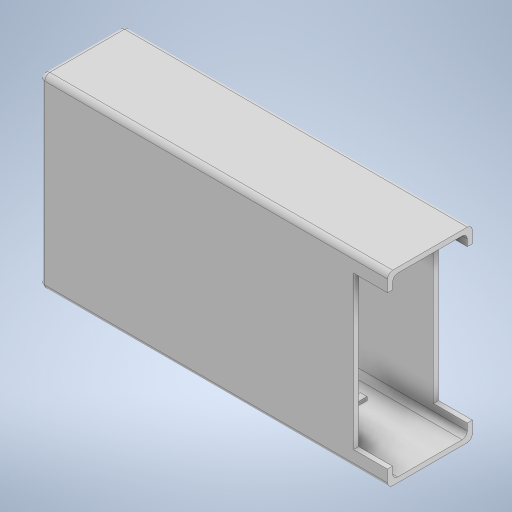
# Autodesk Inventor part: np2_headstage_box_v2
Saved by Autodesk Inventor 2023.3 (Build 273359000, 359)
## iProperties
Created: 2023-11-29
Part Number: np2_headstage_box_v2
Material: Generic
Document SubType Name: Modeling
Designer: mmelin
Density: 1 g/cm^3
Appearance: Default
Author: mmelin
Autodesk Inventor part; units mm, degrees
ref_plane "YZ Plane" through (0, 0, 0) normal (1, 0, 0) x (0, 1, 0)
ref_plane "XZ Plane" through (0, 0, 0) normal (0, 1, 0) x (-1, 0, 0)
ref_plane "XY Plane" through (0, 0, 0) normal (0, 0, 1) x (1, 0, 0)
sketch "Sketch1" plane through (0, 0, 0) normal (0, 0, 1) x (1, 0, 0)
  line L0 (0, 0) -> (18.5, 0)
  line L1 (18.5, 0) -> (18.5, -0.3)
  line L2 (18.5, -0.3) -> (0, -0.3)
  line L3 (0, -0.3) -> (0, 0)
  line L4 (18.5, 10.7) -> (0, 10.7)
  line L5 (0, 10.7) -> (0, 10.4)
  line L6 (0, 10.4) -> (18.5, 10.4)
  line L7 (18.5, 10.4) -> (18.5, 10.7)
  line L8 (0, 10.7) -> (0.3, 10.7)
  line L9 (0.3, 10.7) -> (0.3, -0.3)
  line L10 (0.3, -0.3) -> (0, -0.3)
  line L11 (0, -0.3) -> (0, 10.7)
  point P0 (0.3, 0)
  point P1 (0.3, 10.4)
  dimension "d0" = 0.3
  dimension "d1" = 18.5
  dimension "d2" = 10.4
  dimension "d3" = 0.3
  constraints: 24 end point, 8 parallel, 3 horizontal, 3 perpendicular, 1 collinear, 1 point on line
  measures "d0" distance of L0.end L1.end
  measures "d1" distance of L1.end L2.end
  measures "d2" distance between parallel lines of L0 L6
  measures "d3" distance between parallel lines of L11 L9
extrude "Extrusion1" add sketch "Sketch1" along normal blind 5
sketch "Sketch2" plane through (0.3, 0, 0) normal (1, 0, 0) x (0, 0, -1)
  line L0 (-5, 0) -> (-5, 10.4) projected
  line L1 (0, 0) -> (-5, 0) projected
  line L2 (-5, 10.4) -> (-4.7, 10.4)
  line L3 (-4.7, 10.4) -> (-4.7, 0)
  line L4 (-4.7, 0) -> (-5, 0)
  line L5 (-5, 0) -> (-5, 10.4)
  line L6 (0, 10.4) -> (-5, 10.4) projected
  line L7 (0, 0) -> (-0.3, 0)
  line L8 (-0.3, 0) -> (-0.3, 10.4)
  line L9 (-0.3, 10.4) -> (0, 10.4)
  line L10 (0, 10.4) -> (0, 0)
  point P0 (-0.3, 0)
  dimension "d6" = 0.3
  dimension "d7" = 0.3
  constraints: 16 end point, 4 parallel, 2 horizontal, 2 perpendicular, 2 point on line
  measures "d6" distance between parallel lines of L10 L8
  measures "d7" distance between parallel lines of L0 L3
extrude "Extrusion2" add sketch "Sketch2" along normal up to surface (18.2 mm away) contours L0 L2 L3 L1 | L8 L6 L10 L1
sketch "Sketch3" plane through (0, -0.3, 0) normal (-1, 0, 0) x (0, 0, 1)
  line L0 (0.9, 5.2) -> (3.2, 5.2)
  line L1 (3.2, 5.2) -> (3.2, 7.5)
  line L2 (3.2, 7.5) -> (0.9, 7.5)
  line L3 (0.9, 7.5) -> (0.9, 5.2)
  line L4 (5, 11) -> (5, 0) projected
  line L5 (0, 11) -> (5, 11) projected
  point P0 (0, 0.3)
  dimension "d10" = 2.3
  dimension "d11" = 2.3
  dimension "d12" = 1.8
  dimension "d13" = 3.5
  constraints: 8 end point, 2 parallel, 1 horizontal, 1 perpendicular
  measures "d10" distance of L2.end L0.start
  measures "d11" distance of L1.end L2.end
  measures "d12" distance between parallel lines of L4 L1
  measures "d13" distance between parallel lines of L5 L2
extrude "Extrusion3" cut sketch "Sketch3" against normal up to surface (0.3 mm away)
sketch "Sketch4" plane through (0.3, 0, 0.3) normal (0, 1, 0) x (1, 0, 0)
  line L0 (15, -3.3) -> (15.4, -3.3)
  line L1 (15.4, -3.3) -> (15.4, -1.1)
  line L2 (15.4, -1.1) -> (15, -1.1)
  line L3 (15, -1.1) -> (15, -3.3)
  line L4 (0, 0) -> (0, -4.4) projected
  line L5 (15.4, -3.3) -> (15.4, -4.4) construction
  line L6 (0, -4.4) -> (18.2, -4.4) construction
  line L7 (15.4, -1.1) -> (15.4, 0) construction
  line L8 (18.2, 0) -> (0, 0) construction
  point P0 (-0.3, 0.3)
  dimension "d16" = 15
  dimension "d17" = 0.4
  dimension "d18" = 2.2
  constraints: 12 end point, 2 parallel, 2 perpendicular, 2 point on line, 1 collinear, 1 horizontal, 1 vertical
  measures "d16" distance between parallel lines of L3 L4
  measures "d17" distance between parallel lines of L3 L1
  measures "d18" distance between parallel lines of L0 L2
extrude "Extrusion4" add sketch "Sketch4" along normal blind 0.2
sketch "Sketch5" plane through (0.3, 10.4, 0.3) normal (0, -1, 0) x (1, 0, 0)
  line L0 (15.4, 3.3) -> (15.4, 1.1) projected
  line L1 (15.4, 1.1) -> (15, 1.1) projected
  line L2 (15, 1.1) -> (15, 3.3) projected
  line L3 (15, 3.3) -> (15.4, 3.3) projected
  point P0 (-0.3, -0.3)
extrude "Extrusion5" add sketch "Sketch5" along normal blind 0.2
fillet "Fillet1" radius 0.3 16 edges at (9.25, -0.3, 5) (9.25, -0.3, 0) (0, -0.3, 2.5) (0, 5.2, 0) (0, 5.2, 5) (9.25, 10.7, 5) (9.25, 10.7, 0) (0, 10.7, 2.5) (0.3, 10.4, 2.5) (0.3, 5.2, 4.7) (0.3, 0, 2.5) (0.3, 5.2, 0.3) (9.4, 0, 0.3) (9.4, 0, 4.7) (9.4, 10.4, 0.3) (9.4, 10.4, 4.7)
sketch "Sketch6" plane through (18.5, 0, 0) normal (1, 0, 0) x (0, 0, -1)
  line L0 (-0.3, 10.7) -> (-4.7, 10.7) projected
  arc A0 (-4.7, 10.7) -> (-5, 10.4) centre (-4.7, 10.4) ccw projected
  line L1 (-5, 0) -> (-5, 10.4) projected
  line L2 (-4.7, 10.1) -> (-4.7, 0.3) projected
  arc A1 (-4.4, 10.4) -> (-4.7, 10.1) centre (-4.4, 10.1) ccw projected
  line L3 (-0.6, 10.4) -> (-4.4, 10.4) projected
  arc A2 (0, 10.4) -> (-0.3, 10.7) centre (-0.3, 10.4) ccw projected
  arc A3 (-0.3, 10.1) -> (-0.6, 10.4) centre (-0.6, 10.1) ccw projected
  line L4 (0, 0) -> (0, 10.4) projected
  line L5 (-0.3, 0.3) -> (-0.3, 10.1) projected
  arc A4 (-0.6, 0) -> (-0.3, 0.3) centre (-0.6, 0.3) ccw projected
  arc A5 (-0.3, -0.3) -> (0, 0) centre (-0.3, 0) ccw projected
  line L6 (-0.3, -0.3) -> (-4.7, -0.3) projected
  line L7 (-0.6, 0) -> (-4.4, 0) projected
  arc A6 (-5, 0) -> (-4.7, -0.3) centre (-4.7, 0) ccw projected
  arc A7 (-4.7, 0.3) -> (-4.4, 0) centre (-4.4, 0.3) ccw projected
  line L8 (-5, 9.7) -> (-4.7, 9.7)
  line L9 (-0.3, 9.7) -> (0, 9.7)
  line L10 (-4.7, 10.7) -> (-0.3, 10.7) projected
  line L11 (-4, 10.7) -> (-4, 10.4)
  line L12 (-1, 10.7) -> (-1, 10.4)
  line L13 (-0.3, 0.7) -> (0, 0.7)
  line L14 (0, 10.4) -> (0, 0) projected
  line L15 (-4.7, 0.7) -> (-5, 0.7)
  line L16 (-4, 0) -> (-4, -0.3)
  line L17 (-1, 0) -> (-1, -0.3)
  dimension "d24" = 1
  dimension "d25" = 1
  dimension "d26" = 1
  dimension "d27" = 1
  constraints: 16 end point, 16 point on line, 5 perpendicular, 4 collinear, 2 equal length, 1 horizontal
  measures "d24" distance between parallel lines of L0 L8
  measures "d25" distance between parallel lines of L4 L12
  measures "d26" distance between parallel lines of L1 L11
  measures "d27" distance between parallel lines of L6 L15
extrude "Extrusion6" add sketch "Sketch6" along normal blind 2 contours A2 L4 L9 L5 A3 L3 L12 L0 | L12 L3 L11 L0 | L11 L3 A1 L2 L8 L1 A0 L0 | L4 A5 L6 L17 L7 A4 L5 L13 | L15 L2 A7 L7 L16 L6 A6 L1 | L6 L16 L7 L17
equation "\"d3\" = d0"
equation "\"d7\" = d6"
equation "\"d11\" = d10"
equation "\"d26\" = d25"
body "Solid1"
